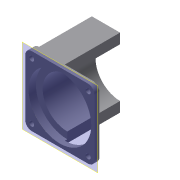
# Autodesk Inventor part: 30_Cube_Z_Focus_MGN_NEMA_Motoradapter_NEMA11_v3
Saved by Autodesk Inventor 2022 (Build 260153000, 153)
## iProperties
Created: 2021-10-20
Part Number: 30_Cube_Z_Focus_MGN_NEMA_Motoradapter_NEMA11_v3
Material: Generic
Document SubType Name: Modeling
Designer: diederichbenedict
Density: 1 g/cm^3
Appearance: Default
Author: diederichbenedict
Autodesk Inventor part; units mm, degrees
ref_plane "YZ Plane" through (0, 0, 0) normal (1, 0, 0) x (0, 1, 0)
ref_plane "XZ Plane" through (0, 0, 0) normal (0, 1, 0) x (-1, 0, 0)
ref_plane "Work Plane3" through (-9.83, 0, 22) normal (0, 0, -1) x (0, -1, 0)
sketch "Sketch2" plane through (-9.83, 0, 22) normal (0, 0, -1) x (0, -1, 0)
  line L0 (14, 11.5) -> (14, -11.5) construction
  arc A0 (14, 11.5) -> (11.5, 14) centre (11.5, 11.5) ccw construction
  line L1 (-11.5, 14) -> (11.5, 14) construction
  arc A1 (-11.5, 14) -> (-14, 11.5) centre (-11.5, 11.5) ccw construction
  line L2 (-14, -11.5) -> (-14, 11.5) construction
  arc A2 (-14, -11.5) -> (-11.5, -14) centre (-11.5, -11.5) ccw construction
  line L3 (11.5, -14) -> (-11.5, -14) construction
  arc A3 (11.5, -14) -> (14, -11.5) centre (11.5, -11.5) ccw construction
  circle A4 centre (0, 0) radius 11 construction
  circle A5 centre (-11.5, 11.5) radius 1.025 construction
  circle A6 centre (11.5, 11.5) radius 1.025 construction
  circle A7 centre (11.5, -11.5) radius 1.025 construction
  circle A8 centre (-11.5, -11.5) radius 1.025 construction
  line L4 (14.1, -11.5) -> (14.1, 11.5)
  arc A9 (14.1, 11.5) -> (11.5, 14.1) centre (11.5, 11.5) ccw
  line L5 (11.5, 14.1) -> (-11.5, 14.1)
  arc A10 (-11.5, 14.1) -> (-14.1, 11.5) centre (-11.5, 11.5) ccw
  line L6 (-14.1, 11.5) -> (-14.1, -11.5)
  arc A11 (-14.1, -11.5) -> (-11.5, -14.1) centre (-11.5, -11.5) ccw
  line L7 (-11.5, -14.1) -> (11.5, -14.1)
  arc A12 (11.5, -14.1) -> (14.1, -11.5) centre (11.5, -11.5) ccw
  circle A13 centre (0, 0) radius 12.75
  circle A14 centre (-11.5, -11.5) radius 1.025
  circle A15 centre (11.5, -11.5) radius 1.025
  circle A16 centre (11.5, 11.5) radius 1.025
  circle A17 centre (-11.5, 11.5) radius 1.025
  point P0 (0, -9.83)
  dimension "d3" = 0.1
  dimension "d4" = 25.5
  dimension "d5" = 0
  dimension "d6" = 0
  dimension "d7" = 0
  dimension "d8" = 0
  constraints: 9 centre point, 8 end point, 8 point on circle, 1 coincident, 7 other
  measures "d3" radial gap between concentric circles of A3 A12
  measures "d4" diameter of A13
  measures "d5" radial gap between concentric circles of A8 A14
  measures "d6" radial gap between concentric circles of A7 A15
  measures "d7" radial gap between concentric circles of A6 A16
  measures "d8" radial gap between concentric circles of A5 A17
extrude "Extrusion2" add sketch "Sketch2" along normal blind 3
sketch "Sketch3" plane through (-9.83, 0, 19) normal (0, 0, -1) x (-1, 0, 0)
  circle A0 centre (0, 0) radius 12.75 projected
  circle A1 centre (11.5, 11.5) radius 1.025 projected
  circle A2 centre (11.5, -11.5) radius 1.025 projected
  circle A3 centre (-11.5, -11.5) radius 1.025 projected
  circle A4 centre (-11.5, 11.5) radius 1.025 projected
  line L0 (-11.5, -14.1) -> (11.5, -14.1) projected
  arc A5 (11.5, -14.1) -> (14.1, -11.5) centre (11.5, -11.5) ccw projected
  line L1 (14.1, -11.5) -> (14.1, 11.5) projected
  arc A6 (14.1, 11.5) -> (11.5, 14.1) centre (11.5, 11.5) ccw projected
  line L2 (11.5, 14.1) -> (-11.5, 14.1) projected
  arc A7 (-11.5, 14.1) -> (-14.1, 11.5) centre (-11.5, 11.5) ccw projected
  line L3 (-14.1, 11.5) -> (-14.1, -11.5) projected
  arc A8 (-14.1, -11.5) -> (-11.5, -14.1) centre (-11.5, -11.5) ccw projected
  line L4 (-11.5, -14.1) -> (11.5, -14.1) projected
  line L5 (0, -14.1) -> (0, -12.75)
  line L6 (0, 12.75) -> (0, 14.1)
  line L7 (11.5, 14.1) -> (-11.5, 14.1) projected
  circle A9 centre (0, 0) radius 10
  line L8 (0, -10) -> (0, -12.75)
  line L9 (0, 10) -> (0, 12.75)
  point P0 (-9.83, 0)
  dimension "d11" = 20
  constraints: 8 end point, 4 point on circle, 2 collinear, 2 midpoint, 2 point on line, 1 centre point, 1 coincident, 1 perpendicular
  measures "d11" diameter of A9
ref_plane "Work Plane4" through (-37.83, -24.85, 0) normal (0, 0, -1) x (0, 1, 0)
extrude "Extrusion3" add sketch "Sketch3" along normal blind 21.5 contours A0 L8 A9 L9 | A0 L6 L2 A6 L1 A5 L0 L5 picked at (11.7268, -0.9457)
sketch "Sketch4" plane through (-9.83, -14.1, -2.5) normal (0, 0, -1) x (-1, 0, 0)
  circle A0 centre (4.2632, 2.351) radius 1.4
  circle A1 centre (11.5541, 7.5847) radius 1.4
  arc A2 (0, 4.1) -> (0, 24.1) centre (0, 14.1) ccw projected
  line L0 (10, 14.1) -> (14.0989, 14.1)
  circle A3 centre (4.2632, 25.849) radius 1.4
  circle A4 centre (11.5541, 20.6153) radius 1.4
  point P0 (-9.83, 14.1)
  dimension "d16" = 2.8
  dimension "d17" = 2.8
  constraints: 4 centre point, 2 end point, 2 symmetric about line, 1 horizontal, 1 point on circle, 2 other
  measures "d16" diameter of A0
  measures "d17" diameter of A1
extrude "Extrusion4" cut sketch "Sketch4" against normal blind 15
sketch "Sketch5" plane through (-9.83, -14.1, -2.5) normal (0, 0, -1) x (-1, 0, 0)
  circle A0 centre (11.5, 2.6) radius 1.025 projected
  circle A1 centre (11.5, 25.6) radius 1.025 projected
  circle A2 centre (11.5, 2.6) radius 2.6
  circle A3 centre (11.5, 25.6) radius 2.6
  point P0 (-9.83, 14.1)
  point P1 (14.1, 2.6)
  dimension "d11" = 20
  constraints: 2 coincident, 1 centre point, 1 horizontal alignment, 2 other
extrude "Extrusion5" cut sketch "Sketch5" against normal up to surface (21.5 mm away) contours A0 | A1 | A2 | A3
sketch "Sketch6" plane through (-9.83, 0, 19) normal (0, 0, -1) x (-1, 0, 0)
  circle A0 centre (-11.5, 11.5) radius 1.025 projected
  circle A1 centre (-11.5, -11.5) radius 1.025 projected
  line L0 (0, -14.1) -> (0, -12.75) projected
  arc A2 (0, 12.75) -> (0, -12.75) centre (0, 0) ccw projected
  line L1 (0, 12.75) -> (0, 14.1) projected
  line L2 (0, 14.1) -> (-11.5, 14.1) projected
  arc A3 (-11.5, 14.1) -> (-14.1, 11.5) centre (-11.5, 11.5) ccw projected
  line L3 (-14.1, 11.5) -> (-14.1, -11.5) projected
  arc A4 (-14.1, -11.5) -> (-11.5, -14.1) centre (-11.5, -11.5) ccw projected
  line L4 (-11.5, -14.1) -> (0, -14.1) projected
  point P0 (-9.83, 0)
extrude "Extrusion6" cut sketch "Sketch6" against normal blind 1
body "Solid2"
